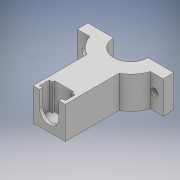
# Autodesk Inventor part: prism_holder_1
Saved by Autodesk Inventor 2018 (Build 220112000, 112)
## iProperties
Created: 2017-11-13
Part Number: prism_holder_1
Material: Generic
Document SubType Name: Modeling
Designer: Bardo91
Density: 1 g/cm^3
Appearance: Default
Author: Bardo91
Autodesk Inventor part; units mm, degrees
ref_plane "YZ Plane" through (0, 0, 0) normal (1, 0, 0) x (0, 1, 0)
ref_plane "XZ Plane" through (0, 0, 0) normal (0, 1, 0) x (-1, 0, 0)
ref_plane "XY Plane" through (0, 0, 0) normal (0, 0, 1) x (1, 0, 0)
sketch "Sketch1" plane through (0, 0, 0) normal (0, 0, 1) x (1, 0, 0)
  line L0 (0, 0) -> (15, 0)
  line L1 (15, 0) -> (15, 30)
  line L2 (15, 30) -> (0, 30)
  line L3 (0, 30) -> (0, 0)
  line L4 (7.5, 30) -> (7.5, 38)
  arc A0 (-0.5, 38) -> (15.5, 38) centre (7.5, 38) ccw
  arc A1 (-7.5, 38) -> (22.5, 38) centre (7.5, 38) ccw
  line L5 (-0.5, 38) -> (-7.5, 38)
  line L6 (15.5, 38) -> (22.5, 38)
  line L7 (22.5, 38) -> (27.5, 38)
  line L8 (27.5, 38) -> (27.5, 33)
  line L9 (27.5, 33) -> (21.6421, 33)
  line L10 (-7.5, 38) -> (-12.5, 38)
  line L11 (-12.5, 38) -> (-12.5, 33)
  line L12 (-12.5, 33) -> (-6.6421, 33)
  dimension "d0" = 15
  dimension "d1" = 30
  dimension "d2" = 8
  dimension "d3" = 16
  dimension "d4" = 30
  dimension "d5" = 5
  dimension "d6" = 5
  dimension "d7" = 5
  dimension "d8" = 5
  constraints: 26 end point, 6 point on circle, 5 perpendicular, 5 point on line, 2 centre point, 2 coincident, 1 horizontal, 1 midpoint, 1 vertical
  measures "d0" distance of L0.start L0.end
  measures "d1" distance of L0.end L1.end
  measures "d2" distance of L4.start L4.end
  measures "d3" diameter of A0
  measures "d4" diameter of A1
  measures "d5" distance of L6.end L7.end
  measures "d6" distance of L7.end L8.end
  measures "d7" distance of L5.end L10.end
  measures "d8" distance of L10.end L11.end
extrude "Extrusion1" add sketch "Sketch1" along normal blind 15
sketch "Sketch2" plane through (0, 0, 15) normal (0, 0, 1) x (1, 0, 0)
  line L0 (0, 0) -> (15, 0) projected
  line L1 (7.5, 0) -> (3, 0)
  line L2 (3, 0) -> (3, 1.5)
  line L3 (3, 1.5) -> (1.5, 1.5)
  line L4 (1.5, 1.5) -> (1.5, 6)
  line L5 (1.5, 6) -> (3, 6)
  line L6 (3, 6) -> (3, 7)
  line L7 (7.5, 0) -> (12, 0)
  line L8 (12, 0) -> (12, 1.5)
  line L9 (12, 1.5) -> (13.5, 1.5)
  line L10 (13.5, 1.5) -> (13.5, 6)
  line L11 (13.5, 6) -> (12, 6)
  line L12 (12, 6) -> (12, 7)
  line L13 (12, 7) -> (3, 7)
  dimension "d11" = 4.5
  dimension "d12" = 1.5
  dimension "d13" = 1.5
  dimension "d14" = 4.5
  dimension "d15" = 1.5
  dimension "d16" = 1
  dimension "d17" = 4.5
  dimension "d18" = 1.5
  constraints: 26 end point, 6 perpendicular, 4 point on line, 2 horizontal, 2 vertical, 1 midpoint
  measures "d11" distance of L1.start L1.end
  measures "d12" distance of L1.end L2.end
  measures "d13" distance of L2.end L3.end
  measures "d14" distance of L3.end L4.end
  measures "d15" distance of L4.end L5.end
  measures "d16" distance of L5.end L6.end
  measures "d17" distance of L1.start L7.end
  measures "d18" distance of L8.end L9.end
sketch "Sketch3" plane through (0, 0, 0) normal (0, -1, 0) x (1, 0, 0)
  line L0 (-0.5, 15) -> (15.5, 15) projected
  line L1 (7.5, 15) -> (7.5, 7.5)
  circle A0 centre (7.5, 7.5) radius 4.5
  point P0 (0, 0)
  dimension "d19" = 7.5
  dimension "d20" = 9
  constraints: 2 end point, 1 centre point, 1 coincident, 1 midpoint, 1 vertical
  measures "d19" distance of L1.start L1.end
  measures "d20" diameter of A0
extrude "Extrusion2" cut sketch "Sketch3" against normal blind 1.5
sketch "Sketch4" plane through (7.5, 1.5, 7.5) normal (0, -1, 0) x (1, 0, 0)
  point P0 (-7.5, -7.5)
extrude "Extrusion3" cut sketch "Sketch2" against normal blind 7.5
sketch "Sketch5" plane through (0, 0, 7.5) normal (0, 0, 1) x (1, 0, 0)
  line L0 (13.5, 6) -> (13.5, 1.5) projected
  line L1 (3, 1.5) -> (1.5, 1.5) projected
  line L2 (13.5, 1.5) -> (1.5, 1.5)
  line L3 (1.5, 1.5) -> (1.5, 6) projected
  line L4 (1.5, 1.5) -> (1.5, 6)
  line L5 (1.5, 6) -> (3, 6) projected
  line L6 (1.5, 6) -> (3, 6)
  line L7 (3, 7) -> (12, 7) projected
  line L8 (3, 6) -> (3, 7)
  line L9 (3, 7) -> (12, 7)
  line L10 (12, 6) -> (13.5, 6) projected
  line L11 (12, 7) -> (12, 6)
  line L12 (12, 6) -> (13.5, 6)
  line L13 (13.5, 6) -> (13.5, 1.5)
  point P0 (0, 0)
  constraints: 16 end point, 4 perpendicular, 2 collinear, 1 horizontal, 1 vertical
extrude "Extrusion4" cut sketch "Sketch5" against normal blind 5
sketch "Sketch6" plane through (-12.5, 38, 0) normal (0, 1, 0) x (1, 0, 0)
  line L0 (0, 0) -> (0, -15) projected
  line L1 (0, -7.5) -> (4, -7.5)
  line L2 (40, 0) -> (40, -15) projected
  line L3 (40, -7.5) -> (36, -7.5)
  circle A0 centre (4, -7.5) radius 1.75
  circle A1 centre (36, -7.5) radius 1.75
  point P0 (12.5, 0)
  dimension "d27" = 4
  dimension "d28" = 4
  dimension "d29" = 3.5
  dimension "d30" = 3.5
  constraints: 4 end point, 2 centre point, 2 coincident, 2 horizontal, 2 midpoint
  measures "d27" distance of L1.start L1.end
  measures "d28" distance of L3.start L3.end
  measures "d29" diameter of A0
  measures "d30" diameter of A1
extrude "Extrusion5" cut sketch "Sketch6" against normal through all
body "Solid1"
